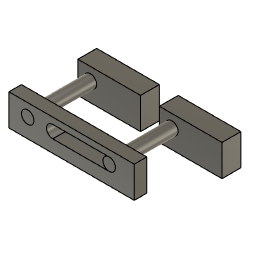
200405_jointExample_pinSlot&Trucks_v2 (Autodesk Fusion 360 design; units mm, degrees)
Autodesk Fusion 360 part; units mm, degrees
sketch "Sketch2" plane through (0, 0, 0) normal (0, 1, 0) x (1, 0, 0) in component "bar"
  line L0 (0, 0) -> (100, 0)
  line L1 (100, 0) -> (100, 25)
  line L2 (100, 25) -> (0, 25)
  line L3 (0, 25) -> (0, 0)
  circle A0 centre (15, 10) radius 5
  line L4 (35, 5) -> (80, 5)
  arc A1 (80, 5) -> (80, 15) centre (80, 10) ccw
  line L5 (80, 15) -> (35, 15)
  arc A2 (35, 15) -> (35, 5) centre (35, 10) ccw
  line L6 (35, 10) -> (80, 10) construction
  dimension "d9" = 0
  dimension "d10" = 0
  dimension "d11" = 0
  dimension "d12" = 0
  constraint horizontal L0
  constraint vertical L1
  constraint horizontal L2
  constraint vertical L3
  constraint coincident L0.start L3.end
  constraint tangent L4 A1
  constraint tangent A1 L5
  constraint parallel L4 L5
  constraint tangent L5 A2
  constraint tangent L4 A2
  constraint horizontal L6
extrude "Extrude1" add sketch "Sketch2" along normal blind 10 makes body 1 in component "bar"
sketch "Sketch1" plane through (0, 0, 0) normal (0, 1, 0) x (1, 0, 0) in component "rod"
  circle A0 centre (-50, -50) radius 5
  dimension "d5" = 0
  dimension "d6" = 0
  dimension "d7" = 0
  dimension "d8" = 0
  dimension "d43" = 0
  dimension "d44" = 0
  dimension "d45" = 0
  dimension "d46" = 0
extrude "Extrude1'" add sketch "Sketch1" against normal blind 70 separate body makes body 2 in component "rod"
sketch "Sketch1 (2)" plane through (0, 0, 0) normal (0, 1, 0) x (1, 0, 0) in component "truck"
  line L0 (-50, -50) -> (0, -50)
  line L1 (0, -50) -> (0, -25)
  line L2 (0, -25) -> (-50, -25)
  line L3 (-50, -25) -> (-50, -50)
  circle A0 centre (-40, -40) radius 5
  dimension "d39" = 0
  dimension "d40" = 0
  dimension "d41" = 0
  dimension "d42" = 0
  constraint horizontal L0
  constraint vertical L1
  constraint horizontal L2
  constraint vertical L3
extrude "Extrude1''" add sketch "Sketch1 (2)" along normal blind 15 separate body makes body 3 in component "truck"
component "bar" placed x (1, 0, 0) y (0, 1, 0) z (0, 0, 1) at (0, 0, 0)
component "rod" placed x (1, 0, 0) y (0, 1, 0) z (0, 0, 1) at (65, 70, -60)
component "rod" placed x (1, 0, 0) y (0, 1, 0) z (0, 0, 1) at (130, 70, -60)
component "truck" placed x (1, 0, 0) y (0, 1, 0) z (0, 0, 1) at (55, 55, -50)
component "truck" placed x (1, 0, 0) y (0, 1, 0) z (0, 0, 1) at (120, 55, -50)
